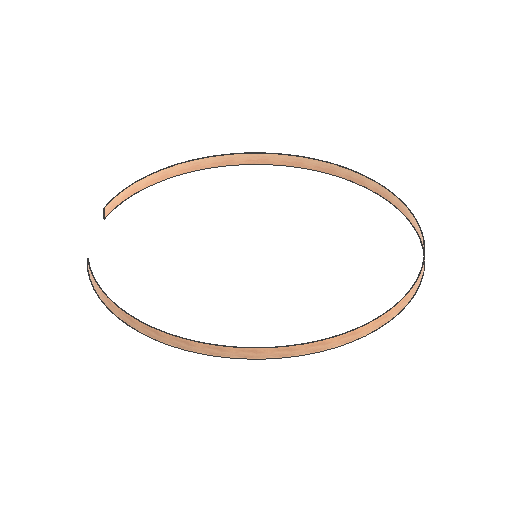
# Autodesk Inventor part: Edge Band - Platform E
Saved by Autodesk Inventor 2021 (Build 250183000, 183)
## iProperties
Created: 2020-05-12
Part Number: Edge Band - Platform E
Material: Wood (Birch)
Document SubType Name: Modeling
Designer: Dan Wikman
Density: 0.55 g/cm^3
Appearance: Birch - Natural Polished
Mass: 1544.34 g
Surface Area: 14609.1 cm^2
Volume: 2807.89 cm^3
Author: Dan Wikman
Autodesk Inventor part; units mm, degrees
ref_plane "YZ Plane" through (0, 0, 0) normal (1, 0, 0) x (0, 1, 0)
ref_plane "XZ Plane" through (0, 0, 0) normal (0, 1, 0) x (-1, 0, 0)
ref_plane "XY Plane" through (0, 0, 0) normal (0, 0, 1) x (1, 0, 0)
sketch "Sketch1" plane through (0, 0, 0) normal (0, 1, 0) x (-1, 0, 0)
  circle A0 centre (0, 0) radius 1218.61
  circle A1 centre (0, 0) radius 1222.61
  dimension "d8" = 2437.22
  dimension "d9" = 2445.22
  constraints: 2 centre point, 2 coincident
  measures "d8" diameter of A0
  measures "d9" diameter of A1
extrude "Extrusion1" add sketch "Sketch1" along normal blind 100
sketch "Sketch2" plane through (0, 100, 0) normal (0, 1, 0) x (1, 0, 0)
  line L0 (-1151.8101, -397.9133) -> (-847.1895, -240.286) projected
  line L1 (-532.3767, -700.7595) -> (-789.8087, -927.3932) projected
  circle A0 centre (0, 0) radius 1222.61 projected
  line L2 (-1155.4034, -399.7726) -> (-1151.8101, -397.9133)
  circle A1 centre (0, 0) radius 1218.61 projected
  line L3 (-793.2013, -930.38) -> (-790.1679, -927.7095)
  point P0 (-1151.8134, -397.915)
  constraints: 4 end point, 2 point on circle, 2 other
extrude "Extrusion2" cut sketch "Sketch2" against normal blind 100 contours L2 A1 L3 A0 picked at (-1147.6869, -413.0424)
body "Solid1"
